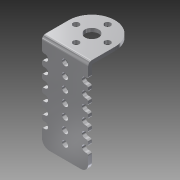
# Autodesk Inventor part: Motor Mount Bracket
Saved by Autodesk Inventor 2015 (Build 190159000, 159)
## iProperties
Created: 2015-10-10
Part Number: Motor Mount Bracket
Material: Aluminum 6061-AHC
Document SubType Name: Modeling
Designer: James
Density: 2.7 g/cm^3
Appearance: Aluminum - Dark
Author: James
Autodesk Inventor part; units mm, degrees
ref_plane "YZ Plane" through (0, 0, 0) normal (1, 0, 0) x (0, 1, 0)
ref_plane "XZ Plane" through (0, 0, 0) normal (0, 1, 0) x (-1, 0, 0)
ref_plane "XY Plane" through (0, 0, 0) normal (0, 0, 1) x (1, 0, 0)
sketch "Sketch1" plane through (0, 0, 0) normal (0, 1, 0) x (-1, 0, 0)
  line L0 (-12.5, 26) -> (12.5, 26)
  line L1 (12.5, 26) -> (12.5, 19.2)
  line L2 (8.5, -26) -> (-8.5, -26)
  circle A0 centre (0, 19.6) radius 1.65
  line L3 (0, 26) -> (10.85, 26)
  arc A1 (10.85, 18.2) -> (10.85, 14.8) centre (10.85, 16.5) ccw
  line L4 (10.85, 18.2) -> (11.5, 18.2)
  line L5 (10.85, 14.8) -> (11.5, 14.8)
  arc A2 (11.5, 18.2) -> (12.5, 19.2) centre (11.5, 19.2) ccw
  arc A3 (12.5, 13.8) -> (11.5, 14.8) centre (11.5, 13.8) ccw
  arc A4 (10.85, 11.85) -> (10.85, 8.45) centre (10.85, 10.15) ccw
  line L6 (10.85, 11.85) -> (11.5, 11.85)
  line L7 (10.85, 8.45) -> (11.5, 8.45)
  arc A5 (11.5, 11.85) -> (12.5, 12.85) centre (11.5, 12.85) ccw
  arc A6 (12.5, 7.45) -> (11.5, 8.45) centre (11.5, 7.45) ccw
  arc A7 (10.85, 5.5) -> (10.85, 2.1) centre (10.85, 3.8) ccw
  line L8 (10.85, 5.5) -> (11.5, 5.5)
  line L9 (10.85, 2.1) -> (11.5, 2.1)
  arc A8 (11.5, 5.5) -> (12.5, 6.5) centre (11.5, 6.5) ccw
  arc A9 (12.5, 1.1) -> (11.5, 2.1) centre (11.5, 1.1) ccw
  arc A10 (10.85, -0.85) -> (10.85, -4.25) centre (10.85, -2.55) ccw
  line L10 (10.85, -0.85) -> (11.5, -0.85)
  line L11 (10.85, -4.25) -> (11.5, -4.25)
  arc A11 (11.5, -0.85) -> (12.5, 0.15) centre (11.5, 0.15) ccw
  arc A12 (12.5, -5.25) -> (11.5, -4.25) centre (11.5, -5.25) ccw
  arc A13 (10.85, -7.2) -> (10.85, -10.6) centre (10.85, -8.9) ccw
  line L12 (10.85, -7.2) -> (11.5, -7.2)
  line L13 (10.85, -10.6) -> (11.5, -10.6)
  arc A14 (11.5, -7.2) -> (12.5, -6.2) centre (11.5, -6.2) ccw
  arc A15 (12.5, -11.6) -> (11.5, -10.6) centre (11.5, -11.6) ccw
  arc A16 (10.85, -13.55) -> (10.85, -16.95) centre (10.85, -15.25) ccw
  line L14 (10.85, -13.55) -> (11.5, -13.55)
  line L15 (10.85, -16.95) -> (11.5, -16.95)
  arc A17 (11.5, -13.55) -> (12.5, -12.55) centre (11.5, -12.55) ccw
  arc A18 (12.5, -17.95) -> (11.5, -16.95) centre (11.5, -17.95) ccw
  line L16 (12.5, 13.8) -> (12.5, 12.85)
  line L17 (12.5, 7.45) -> (12.5, 6.5)
  line L18 (12.5, 1.1) -> (12.5, 0.15)
  line L19 (12.5, -5.25) -> (12.5, -6.2)
  line L20 (12.5, -11.6) -> (12.5, -12.55)
  line L21 (12.5, -17.95) -> (12.5, -22)
  line L22 (-12.5, 26) -> (-12.5, 19.2)
  arc A19 (-10.85, 14.8) -> (-10.85, 18.2) centre (-10.85, 16.5) ccw
  line L23 (-10.85, 18.2) -> (-11.5, 18.2)
  line L24 (-10.85, 14.8) -> (-11.5, 14.8)
  arc A20 (-12.5, 19.2) -> (-11.5, 18.2) centre (-11.5, 19.2) ccw
  arc A21 (-11.5, 14.8) -> (-12.5, 13.8) centre (-11.5, 13.8) ccw
  arc A22 (-11.5, 8.45) -> (-12.5, 7.45) centre (-11.5, 7.45) ccw
  line L25 (-10.85, 8.45) -> (-11.5, 8.45)
  line L26 (-10.85, 11.85) -> (-11.5, 11.85)
  arc A23 (-12.5, 12.85) -> (-11.5, 11.85) centre (-11.5, 12.85) ccw
  arc A24 (-10.85, 8.45) -> (-10.85, 11.85) centre (-10.85, 10.15) ccw
  arc A25 (-11.5, 2.1) -> (-12.5, 1.1) centre (-11.5, 1.1) ccw
  line L27 (-10.85, 2.1) -> (-11.5, 2.1)
  line L28 (-10.85, 5.5) -> (-11.5, 5.5)
  arc A26 (-12.5, 6.5) -> (-11.5, 5.5) centre (-11.5, 6.5) ccw
  arc A27 (-10.85, 2.1) -> (-10.85, 5.5) centre (-10.85, 3.8) ccw
  arc A28 (-11.5, -4.25) -> (-12.5, -5.25) centre (-11.5, -5.25) ccw
  line L29 (-10.85, -4.25) -> (-11.5, -4.25)
  line L30 (-10.85, -0.85) -> (-11.5, -0.85)
  arc A29 (-12.5, 0.15) -> (-11.5, -0.85) centre (-11.5, 0.15) ccw
  arc A30 (-10.85, -4.25) -> (-10.85, -0.85) centre (-10.85, -2.55) ccw
  arc A31 (-11.5, -10.6) -> (-12.5, -11.6) centre (-11.5, -11.6) ccw
  line L31 (-10.85, -10.6) -> (-11.5, -10.6)
  line L32 (-10.85, -7.2) -> (-11.5, -7.2)
  arc A32 (-12.5, -6.2) -> (-11.5, -7.2) centre (-11.5, -6.2) ccw
  arc A33 (-10.85, -10.6) -> (-10.85, -7.2) centre (-10.85, -8.9) ccw
  arc A34 (-11.5, -16.95) -> (-12.5, -17.95) centre (-11.5, -17.95) ccw
  line L33 (-10.85, -16.95) -> (-11.5, -16.95)
  line L34 (-10.85, -13.55) -> (-11.5, -13.55)
  arc A35 (-12.5, -12.55) -> (-11.5, -13.55) centre (-11.5, -12.55) ccw
  arc A36 (-10.85, -16.95) -> (-10.85, -13.55) centre (-10.85, -15.25) ccw
  line L35 (-12.5, 13.8) -> (-12.5, 12.85)
  line L36 (-12.5, 7.45) -> (-12.5, 6.5)
  line L37 (-12.5, 1.1) -> (-12.5, 0.15)
  line L38 (-12.5, -5.25) -> (-12.5, -6.2)
  line L39 (-12.5, -11.6) -> (-12.5, -12.55)
  line L40 (-12.5, -17.95) -> (-12.5, -22)
  arc A37 (8.5, -26) -> (12.5, -22) centre (8.5, -22) ccw
  arc A38 (-12.5, -22) -> (-8.5, -26) centre (-8.5, -22) ccw
  circle A39 centre (0, 13.25) radius 1.65
  circle A40 centre (0, 6.9) radius 1.65
  circle A41 centre (0, 0.55) radius 1.65
  circle A42 centre (0, -5.8) radius 1.65
  circle A43 centre (0, -12.15) radius 1.65
  circle A44 centre (0, -18.5) radius 1.65
  point P0 (-12.5, -26)
  point P1 (12.5, -26)
  point P2 (12.5, 14.8)
  point P3 (12.5, 8.45)
  point P4 (12.5, 2.1)
  point P5 (12.5, -4.25)
  point P6 (12.5, -10.6)
  point P7 (12.5, -16.95)
  point P8 (-12.5, 14.8)
  point P9 (-12.5, 8.45)
  point P10 (-12.5, 2.1)
  point P11 (-12.5, -4.25)
  point P12 (-12.5, -10.6)
  point P13 (-12.5, -16.95)
  dimension "d0" = 52
  dimension "d1" = 25
  dimension "d3" = 3.3
  dimension "d16" = 10.85
  dimension "d18" = 1.7
  dimension "d19" = 1
  dimension "d20" = 1
  dimension "d22" = 1.7
  dimension "d23" = 1
  dimension "d24" = 1
  dimension "d26" = 1.7
  dimension "d27" = 1
  dimension "d28" = 1
  dimension "d30" = 1.7
  dimension "d31" = 1
  dimension "d32" = 1
  dimension "d34" = 1.7
  dimension "d35" = 1
  dimension "d36" = 1
  dimension "d38" = 1.7
  dimension "d39" = 1
  dimension "d40" = 1
  dimension "d42" = 4
  dimension "d44" = 3.3
  dimension "d46" = 3.3
  dimension "d48" = 3.3
  dimension "d50" = 3.3
  dimension "d52" = 3.3
  dimension "d54" = 3.3
  constraints: 82 end point, 76 point on circle, 45 centre point, 21 point on line, 18 tangent, 5 collinear, 2 perpendicular, 1 equal radius, 1 midpoint, 1 parallel, 1 vertical
  measures "d0" distance of point (-12.5, -26) L0.start
  measures "d1" distance of L0.start L0.end
  measures "d3" diameter of A0
  measures "d16" distance of L3.start L3.end
  measures "d18" radius of A1
  measures "d19" radius of A2
  measures "d20" radius of A3
  measures "d22" radius of A4
  measures "d23" radius of A5
  measures "d24" radius of A6
  measures "d26" radius of A7
  measures "d27" radius of A8
  measures "d28" radius of A9
  measures "d30" radius of A10
  measures "d31" radius of A11
  measures "d32" radius of A12
  measures "d34" radius of A13
  measures "d35" radius of A14
  measures "d36" radius of A15
  measures "d38" radius of A16
  measures "d39" radius of A17
  measures "d40" radius of A18
  measures "d42" radius of A37
  measures "d44" diameter of A39
  measures "d46" diameter of A40
  measures "d48" diameter of A41
  measures "d50" diameter of A42
  measures "d52" diameter of A43
  measures "d54" diameter of A44
extrude "Extrusion1" add sketch "Sketch1" along normal blind 2
sketch "Sketch2" plane through (0, 2, 0) normal (0, 1, 0) x (1, 0, 0)
  line L0 (-12.5, -26) -> (12.5, -26)
  line L1 (12.5, -26) -> (12.5, -24)
  line L2 (12.5, -24) -> (-12.5, -24)
  line L3 (-12.5, -24) -> (-12.5, -26)
  point P0 (0, 0)
  dimension "d60" = 2
  constraints: 8 end point, 2 parallel, 1 horizontal, 1 perpendicular
  measures "d60" distance of L1.end L0.end
extrude "Extrusion2" add sketch "Sketch2" along normal blind 27
sketch "Sketch3" plane through (-12.5, 0, 26) normal (0, 0, 1) x (1, 0, 0)
  circle A0 centre (12.5, 14.5) radius 3.75
  circle A1 centre (12.5, 23) radius 1.65
  circle A2 centre (4, 14.5) radius 1.65
  circle A3 centre (12.5, 6) radius 1.65
  circle A4 centre (21, 14.5) radius 1.65
  line L0 (0, 0) -> (0, 29) projected
  arc A5 (25, 14.5) -> (0, 14.5) centre (12.5, 14.5) ccw
  line L1 (0, 14.5) -> (0, 29)
  line L2 (0, 29) -> (25, 29)
  line L3 (25, 29) -> (25, 14.5)
  point P0 (12.5, 0)
  dimension "d63" = 14.5
  dimension "d64" = 7.5
  dimension "d66" = 3.3
  dimension "d69" = 360
  constraints: 6 centre point, 6 end point, 2 coincident, 2 point on circle, 1 horizontal, 1 midpoint, 1 perpendicular, 1 tangent, 1 vertical, 9 other
  measures "d63" distance of point (12.5, 0) point (12.5, 14.5)
  measures "d64" diameter of A0
  measures "d66" diameter of A1
extrude "Extrusion3" cut sketch "Sketch3" against normal through all
fillet "Fillet1" radius 2 1 edges at (0, 0, 26)
body "Solid1"
